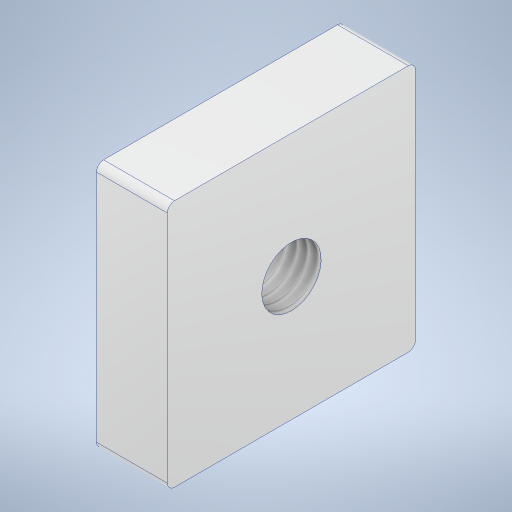
# Autodesk Inventor part: Traversen_Deckel
Saved by Autodesk Inventor 2024.4 (Build 284460000, 460)
## iProperties
Created: 2026-01-10
Part Number: Traversen_Deckel
Material: Aluminium 6061
Description: Traversen_Deckel
Document SubType Name: Modeling
Designer: julia
Mass: 31.5641 g
Surface Area: 39.8405 cm^2
Volume: 11.6904 cm^3
Density: 2.7 g/cm^3
Appearance: Aluminium - flach
DocNumber: Traversen_Deckel.ipt
Folder: I60-Konstruktion\I60-Gruppe-7\Gestell\
VDS_Category: Konstruktion
Masse[kg]: 0,012 kg
Autodesk Inventor part; units mm, degrees
ref_plane "YZ Plane" through (0, 0, 0) normal (1, 0, 0) x (0, 1, 0)
ref_plane "XZ Plane" through (0, 0, 0) normal (0, 1, 0) x (-1, 0, 0)
ref_plane "XY Plane" through (0, 0, 0) normal (0, 0, 1) x (1, 0, 0)
sketch "Skizze1" plane through (0, 0, 0) normal (1, 0, 0) x (0, 1, 0)
  line L0 (-16.5, 17.5) -> (16.5, 17.5)
  line L1 (17.5, 16.5) -> (17.5, -16.5)
  line L2 (16.5, -17.5) -> (-16.5, -17.5)
  line L3 (-17.5, -16.5) -> (-17.5, 16.5)
  line L4 (-17.5, 17.5) -> (17.5, -17.5) construction
  line L5 (17.5, 17.5) -> (-17.5, -17.5) construction
  arc A0 (17.5, 16.5) -> (16.5, 17.5) centre (16.5, 16.5) ccw
  arc A1 (-16.5, 17.5) -> (-17.5, 16.5) centre (-16.5, 16.5) ccw
  arc A2 (-17.5, -16.5) -> (-16.5, -17.5) centre (-16.5, -16.5) ccw
  arc A3 (16.5, -17.5) -> (17.5, -16.5) centre (16.5, -16.5) ccw
  point P0 (0, 0)
  dimension "d0" = 35
  dimension "d1" = 35
  dimension "d2" = 1
  constraints: 12 end point, 8 point on circle, 8 point on line, 8 tangent, 4 centre point, 3 equal radius, 2 midpoint, 2 parallel, 1 horizontal, 1 perpendicular
  measures "d0" distance of L4.end L5.end
  measures "d1" distance of L5.start L4.end
  measures "d2" radius of A0
extrude "Extrusion1" add sketch "Skizze1" along normal blind 10
sketch "Skizze2" plane through (10, 0, 0) normal (1, 0, 0) x (0, 0, -1)
  line L0 (0, 0) -> (0, 17.5)
  line L1 (16.5, 17.5) -> (-16.5, 17.5) projected
  line L2 (0, 0) -> (17.4918, 0)
  constraints: 4 end point, 1 horizontal, 1 midpoint
hole "Bohrung1" at (10, 0, 0) direction (-1, 0, 0) diameter 8.376 end through all thread size "M10x1.5" class "6H" standard "ISO Metric profile"
